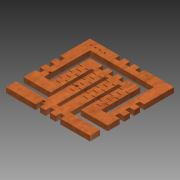
# Autodesk Inventor part: mech
Saved by Autodesk Inventor 2014 SP1 (Build 180222100, 222)
## iProperties
Created: 2015-02-17
Part Number: mech
Material: Wood (Cherry)
Document SubType Name: Modeling
Designer: Erin
Density: 0.63 g/cm^3
Appearance: Cherry - Natural Low Gloss
Author: Erin
Autodesk Inventor part; units mm, degrees
ref_plane "YZ Plane" through (0, 0, 0) normal (1, 0, 0) x (0, 1, 0)
ref_plane "XZ Plane" through (0, 0, 0) normal (0, 1, 0) x (-1, 0, 0)
ref_plane "XY Plane" through (0, 0, 0) normal (0, 0, 1) x (1, 0, 0)
sketch "slots" plane through (0, 0, 0) normal (0, 0, 1) x (1, 0, 0)
  line L0 (61.2067, 31.1821) -> (64.2567, 31.1821)
  line L1 (64.2567, 31.1821) -> (64.2567, 28.1071)
  line L2 (64.2567, 28.1071) -> (61.2067, 28.1071)
  line L3 (61.2067, 28.1071) -> (61.2067, 31.1821)
  line L4 (68.9317, 33.8834) -> (68.9317, 26.9198) construction
  line L5 (67.4067, 31.1821) -> (70.4567, 31.1821)
  line L6 (70.4567, 31.1821) -> (70.4567, 28.1071)
  line L7 (70.4567, 28.1071) -> (67.4067, 28.1071)
  line L8 (67.4067, 28.1071) -> (67.4067, 31.1821)
  line L9 (73.6067, 31.1821) -> (76.6567, 31.1821)
  line L10 (76.6567, 31.1821) -> (76.6567, 28.1071)
  line L11 (76.6567, 28.1071) -> (73.6067, 28.1071)
  line L12 (73.6067, 28.1071) -> (73.6067, 31.1821)
  line L13 (68.9317, 28.1071) -> (68.9317, 27.1937) construction
  point P0 (68.8645, 30.3856)
  dimension "d2" = 3.05
  dimension "d3" = 3.075
  dimension "d99" = 3.15
  dimension "d100" = 3.15
  measures "d2" distance of L1.end L2.end
  measures "d3" distance of L0.end L1.end
  measures "d99" distance between parallel lines of L8 L1
  measures "d100" distance between parallel lines of L12 L6
sketch "flexure" plane through (0, 0, 0) normal (0, 0, 1) x (1, 0, 0)
  line L0 (49.9032, 37.6477) -> (55.9032, 37.6477)
  line L1 (55.9032, 37.6477) -> (55.9032, 19.1477)
  line L2 (55.9032, 19.1477) -> (49.9032, 19.1477)
  line L3 (49.9032, 19.1477) -> (49.9032, 37.6477)
  line L4 (49.9032, 30.1477) -> (52.085, 30.1477)
  line L5 (52.085, 30.1477) -> (52.085, 29.6477)
  line L6 (52.085, 29.6477) -> (49.9032, 29.6477)
  line L7 (49.9032, 29.6477) -> (49.9032, 30.1477)
  line L8 (53.7214, 29.6477) -> (53.7214, 30.1477)
  line L9 (55.9032, 29.6477) -> (53.7214, 29.6477)
  line L10 (53.7214, 30.1477) -> (55.9032, 30.1477)
  line L11 (55.9032, 30.1477) -> (55.9032, 29.6477)
  line L12 (51.5395, 27.1477) -> (54.2668, 27.1477)
  line L13 (54.2668, 27.1477) -> (54.2668, 26.6477)
  line L14 (54.2668, 26.6477) -> (51.5395, 26.6477)
  line L15 (51.5395, 26.6477) -> (51.5395, 27.1477)
  line L16 (49.9032, 28.3977) -> (55.9032, 28.3977) construction
  line L17 (55.9032, 28.3977) -> (49.9032, 28.3977) construction
  line L18 (53.7214, 24.1477) -> (55.9032, 24.1477)
  line L19 (55.9032, 24.1477) -> (55.9032, 23.6477)
  line L20 (55.9032, 23.6477) -> (53.7214, 23.6477)
  line L21 (53.7214, 23.6477) -> (53.7214, 24.1477)
  line L22 (51.5395, 21.1477) -> (54.2668, 21.1477)
  line L23 (54.2668, 21.1477) -> (54.2668, 20.6477)
  line L24 (54.2668, 20.6477) -> (51.5395, 20.6477)
  line L25 (51.5395, 20.6477) -> (51.5395, 21.1477)
  line L26 (49.9032, 24.1477) -> (52.085, 24.1477)
  line L27 (52.085, 24.1477) -> (52.085, 23.6477)
  line L28 (52.085, 23.6477) -> (49.9032, 23.6477)
  line L29 (49.9032, 23.6477) -> (49.9032, 24.1477)
  line L30 (49.9032, 22.3977) -> (55.9032, 22.3977) construction
  line L31 (55.9032, 22.3977) -> (49.9032, 22.3977) construction
  line L32 (53.7214, 36.1477) -> (55.9032, 36.1477)
  line L33 (55.9032, 36.1477) -> (55.9032, 35.6477)
  line L34 (55.9032, 35.6477) -> (53.7214, 35.6477)
  line L35 (53.7214, 35.6477) -> (53.7214, 36.1477)
  line L36 (51.5395, 33.1477) -> (54.2668, 33.1477)
  line L37 (54.2668, 33.1477) -> (54.2668, 32.6477)
  line L38 (54.2668, 32.6477) -> (51.5395, 32.6477)
  line L39 (51.5395, 32.6477) -> (51.5395, 33.1477)
  line L40 (49.9032, 36.1477) -> (52.085, 36.1477)
  line L41 (52.085, 36.1477) -> (52.085, 35.6477)
  line L42 (52.085, 35.6477) -> (49.9032, 35.6477)
  line L43 (49.9032, 35.6477) -> (49.9032, 36.1477)
  line L44 (49.9032, 34.3977) -> (55.9032, 34.3977) construction
  line L45 (55.9032, 34.3977) -> (49.9032, 34.3977) construction
  line L46 (53.7214, 30.1477) -> (55.9032, 30.1477)
  line L47 (55.9032, 30.1477) -> (55.9032, 29.6477)
  line L48 (55.9032, 29.6477) -> (53.7214, 29.6477)
  line L49 (53.7214, 29.6477) -> (53.7214, 30.1477)
  line L50 (51.5395, 27.1477) -> (54.2668, 27.1477)
  line L51 (54.2668, 27.1477) -> (54.2668, 26.6477)
  line L52 (54.2668, 26.6477) -> (51.5395, 26.6477)
  line L53 (51.5395, 26.6477) -> (51.5395, 27.1477)
  line L54 (49.9032, 30.1477) -> (52.085, 30.1477)
  line L55 (52.085, 30.1477) -> (52.085, 29.6477)
  line L56 (52.085, 29.6477) -> (49.9032, 29.6477)
  line L57 (49.9032, 29.6477) -> (49.9032, 30.1477)
  line L58 (49.9032, 28.3977) -> (55.9032, 28.3977) construction
  line L59 (55.9032, 28.3977) -> (49.9032, 28.3977) construction
  line L60 (51.5395, 26.8977) -> (54.2668, 26.8977) construction
  point P0 (52.8239, 25.8216)
  dimension "d22" = 6
  dimension "d24" = 2.1818
  dimension "d27" = 3.8182
  dimension "d32" = 1.6364
  dimension "d33" = 2.7273
  dimension "d41" = 0.5
  dimension "d42" = 0.5
  dimension "d43" = 2.5
  dimension "d93" = 18.5
  dimension "d106" = 6
  dimension "d109" = 6
  dimension "d118" = 10.5
  measures "d22" distance of L1.end L2.end
  measures "d24" distance of L4.start L4.end
  measures "d27" distance of L6.end L9.end
  measures "d32" distance between parallel lines of L15 L3
  measures "d33" distance of L12.start L12.end
  measures "d41" distance of L4.end L5.end
  measures "d42" distance of L12.end L13.end
  measures "d43" distance between parallel lines of L12 L6
  measures "d93" distance of L0.end L1.end
  measures "d106" distance of L10.start L18.start
  measures "d109" distance of L10.start L32.start
  measures "d118" distance between parallel lines of L12 L0
sketch "Sketch1" plane through (0, 0, 0) normal (0, 0, 1) x (1, 0, 0)
  line L0 (-25, 25) -> (25, 25) construction
  line L1 (25, 25) -> (25, -25) construction
  line L2 (25, -25) -> (-25, -25) construction
  line L3 (-25, -25) -> (-25, 25) construction
  line L4 (-25, -25) -> (25, -25)
  line L5 (25, -25) -> (25, -19)
  line L6 (25, -19) -> (-25, -19)
  line L7 (-25, -19) -> (-25, -25)
  line L8 (0, 33.5916) -> (0, -39.9789) construction
  line L9 (-35.9054, 0) -> (42.6007, 0) construction
  line L10 (-25, 25) -> (25, 25)
  line L11 (25, 25) -> (25, 19)
  line L12 (25, 19) -> (-25, 19)
  line L13 (-25, 19) -> (-25, 25)
  line L14 (-25, 19) -> (-19, 19)
  line L15 (-19, 19) -> (-19, -14.5)
  line L16 (-19, -14.5) -> (-25, -14.5)
  line L17 (-25, -14.5) -> (-25, 19)
  line L18 (-19, -14.5) -> (-9, -14.5)
  line L19 (-9, -14.5) -> (-9, -8.5)
  line L20 (-9, -8.5) -> (-19, -8.5)
  line L21 (-19, -8.5) -> (-19, -14.5)
  line L22 (25, 19) -> (19, 19)
  line L23 (19, 19) -> (19, -14.5)
  line L24 (19, -14.5) -> (25, -14.5)
  line L25 (25, -14.5) -> (25, 19)
  line L26 (19, -14.5) -> (9, -14.5)
  line L27 (9, -14.5) -> (9, -8.5)
  line L28 (9, -8.5) -> (19, -8.5)
  line L29 (19, -8.5) -> (19, -14.5)
  line L30 (-15, 15) -> (15, 15)
  line L31 (15, 15) -> (15, 10)
  line L32 (15, 10) -> (-15, 10)
  line L33 (-15, 10) -> (-15, 15)
  line L34 (-7, -8.5) -> (-1, -8.5)
  line L35 (-1, -8.5) -> (-1, -19)
  line L36 (-1, -19) -> (-7, -19)
  line L37 (-7, -19) -> (-7, -8.5)
  line L38 (1, -8.5) -> (7, -8.5)
  line L39 (7, -8.5) -> (7, -19)
  line L40 (7, -19) -> (1, -19)
  line L41 (1, -19) -> (1, -8.5)
  line L42 (-68.1542, 16.5688) -> (-29.44, 16.5688) construction
  line L43 (-29.44, 16.5688) -> (-29.44, -5.0786) construction
  line L44 (-29.44, -5.0786) -> (-68.1542, -5.0786) construction
  line L45 (-68.1542, -5.0786) -> (-68.1542, 16.5688) construction
  circle A0 centre (-21.2866, 22) radius 0.5
  circle A1 centre (-18.6754, 22) radius 0.5
  circle A2 centre (-16, 22) radius 0.5
  circle A3 centre (-13.1389, 22) radius 0.5
  line L46 (-7.725, 25) -> (-4.675, 25)
  line L47 (-4.675, 25) -> (-4.675, 21.925)
  line L48 (-4.675, 21.925) -> (-7.725, 21.925)
  line L49 (-7.725, 21.925) -> (-7.725, 25)
  line L50 (0, 27.7013) -> (0, 20.7377) construction
  line L51 (-1.525, 25) -> (1.525, 25)
  line L52 (1.525, 25) -> (1.525, 21.925)
  line L53 (1.525, 21.925) -> (-1.525, 21.925)
  line L54 (-1.525, 21.925) -> (-1.525, 25)
  line L55 (4.675, 25) -> (7.725, 25)
  line L56 (7.725, 25) -> (7.725, 21.925)
  line L57 (7.725, 21.925) -> (4.675, 21.925)
  line L58 (4.675, 21.925) -> (4.675, 25)
  line L59 (0, 21.925) -> (0, 21.0116) construction
  line L60 (-7.725, -21.925) -> (-4.675, -21.925)
  line L61 (-4.675, -21.925) -> (-4.675, -25)
  line L62 (-4.675, -25) -> (-7.725, -25)
  line L63 (-7.725, -25) -> (-7.725, -21.925)
  line L64 (0, -19.2237) -> (0, -26.1873) construction
  line L65 (-1.525, -21.925) -> (1.525, -21.925)
  line L66 (1.525, -21.925) -> (1.525, -25)
  line L67 (1.525, -25) -> (-1.525, -25)
  line L68 (-1.525, -25) -> (-1.525, -21.925)
  line L69 (4.675, -21.925) -> (7.725, -21.925)
  line L70 (7.725, -21.925) -> (7.725, -25)
  line L71 (7.725, -25) -> (4.675, -25)
  line L72 (4.675, -25) -> (4.675, -21.925)
  line L73 (0, -25) -> (0, -25.9134) construction
  line L74 (-25, -7.725) -> (-25, -4.675)
  line L75 (-25, -4.675) -> (-21.925, -4.675)
  line L76 (-21.925, -4.675) -> (-21.925, -7.725)
  line L77 (-21.925, -7.725) -> (-25, -7.725)
  line L78 (-27.7013, 0) -> (-20.7377, 0) construction
  line L79 (-25, -1.525) -> (-25, 1.525)
  line L80 (-25, 1.525) -> (-21.925, 1.525)
  line L81 (-21.925, 1.525) -> (-21.925, -1.525)
  line L82 (-21.925, -1.525) -> (-25, -1.525)
  line L83 (-25, 4.675) -> (-25, 7.725)
  line L84 (-25, 7.725) -> (-21.925, 7.725)
  line L85 (-21.925, 7.725) -> (-21.925, 4.675)
  line L86 (-21.925, 4.675) -> (-25, 4.675)
  line L87 (-21.925, 0) -> (-21.0116, 0) construction
  line L88 (21.925, -7.725) -> (21.925, -4.675)
  line L89 (21.925, -4.675) -> (25, -4.675)
  line L90 (25, -4.675) -> (25, -7.725)
  line L91 (25, -7.725) -> (21.925, -7.725)
  line L92 (19.2237, 0) -> (26.1873, 0) construction
  line L93 (21.925, -1.525) -> (21.925, 1.525)
  line L94 (21.925, 1.525) -> (25, 1.525)
  line L95 (25, 1.525) -> (25, -1.525)
  line L96 (25, -1.525) -> (21.925, -1.525)
  line L97 (21.925, 4.675) -> (21.925, 7.725)
  line L98 (21.925, 7.725) -> (25, 7.725)
  line L99 (25, 7.725) -> (25, 4.675)
  line L100 (25, 4.675) -> (21.925, 4.675)
  line L101 (25, 0) -> (25.9134, 0) construction
  line L102 (-15, 10) -> (-9, 10)
  line L103 (-9, 10) -> (-9, -8.5)
  line L104 (-9, -8.5) -> (-15, -8.5)
  line L105 (-15, -8.5) -> (-15, 10)
  line L106 (-15, 2.5) -> (-12.8182, 2.5)
  line L107 (-12.8182, 2.5) -> (-12.8182, 2)
  line L108 (-12.8182, 2) -> (-15, 2)
  line L109 (-15, 2) -> (-15, 2.5)
  line L110 (-11.1818, 2) -> (-11.1818, 2.5)
  line L111 (-9, 2) -> (-11.1818, 2)
  line L112 (-11.1818, 2.5) -> (-9, 2.5)
  line L113 (-9, 2.5) -> (-9, 2)
  line L114 (-13.3636, -0.5) -> (-10.6364, -0.5)
  line L115 (-10.6364, -0.5) -> (-10.6364, -1)
  line L116 (-10.6364, -1) -> (-13.3636, -1)
  line L117 (-13.3636, -1) -> (-13.3636, -0.5)
  line L118 (-15, 0.75) -> (-9, 0.75) construction
  line L119 (-9, 0.75) -> (-15, 0.75) construction
  line L120 (-11.1818, -3.5) -> (-9, -3.5)
  line L121 (-9, -3.5) -> (-9, -4)
  line L122 (-9, -4) -> (-11.1818, -4)
  line L123 (-11.1818, -4) -> (-11.1818, -3.5)
  line L124 (-13.3636, -6.5) -> (-10.6364, -6.5)
  line L125 (-10.6364, -6.5) -> (-10.6364, -7)
  line L126 (-10.6364, -7) -> (-13.3636, -7)
  line L127 (-13.3636, -7) -> (-13.3636, -6.5)
  line L128 (-15, -3.5) -> (-12.8182, -3.5)
  line L129 (-12.8182, -3.5) -> (-12.8182, -4)
  line L130 (-12.8182, -4) -> (-15, -4)
  line L131 (-15, -4) -> (-15, -3.5)
  line L132 (-15, -5.25) -> (-9, -5.25) construction
  line L133 (-9, -5.25) -> (-15, -5.25) construction
  line L134 (-11.1818, 8.5) -> (-9, 8.5)
  line L135 (-9, 8.5) -> (-9, 8)
  line L136 (-9, 8) -> (-11.1818, 8)
  line L137 (-11.1818, 8) -> (-11.1818, 8.5)
  line L138 (-13.3636, 5.5) -> (-10.6364, 5.5)
  line L139 (-10.6364, 5.5) -> (-10.6364, 5)
  line L140 (-10.6364, 5) -> (-13.3636, 5)
  line L141 (-13.3636, 5) -> (-13.3636, 5.5)
  line L142 (-15, 8.5) -> (-12.8182, 8.5)
  line L143 (-12.8182, 8.5) -> (-12.8182, 8)
  line L144 (-12.8182, 8) -> (-15, 8)
  line L145 (-15, 8) -> (-15, 8.5)
  line L146 (-15, 6.75) -> (-9, 6.75) construction
  line L147 (-9, 6.75) -> (-15, 6.75) construction
  line L148 (-11.1818, 2.5) -> (-9, 2.5)
  line L149 (-9, 2.5) -> (-9, 2)
  line L150 (-9, 2) -> (-11.1818, 2)
  line L151 (-11.1818, 2) -> (-11.1818, 2.5)
  line L152 (-13.3636, -0.5) -> (-10.6364, -0.5)
  line L153 (-10.6364, -0.5) -> (-10.6364, -1)
  line L154 (-10.6364, -1) -> (-13.3636, -1)
  line L155 (-13.3636, -1) -> (-13.3636, -0.5)
  line L156 (-15, 2.5) -> (-12.8182, 2.5)
  line L157 (-12.8182, 2.5) -> (-12.8182, 2)
  line L158 (-12.8182, 2) -> (-15, 2)
  line L159 (-15, 2) -> (-15, 2.5)
  line L160 (-15, 0.75) -> (-9, 0.75) construction
  line L161 (-9, 0.75) -> (-15, 0.75) construction
  line L162 (-13.3636, -0.75) -> (-10.6364, -0.75) construction
  line L163 (9, 10) -> (15, 10)
  line L164 (15, 10) -> (15, -8.5)
  line L165 (15, -8.5) -> (9, -8.5)
  line L166 (9, -8.5) -> (9, 10)
  line L167 (9, 2.5) -> (11.1818, 2.5)
  line L168 (11.1818, 2.5) -> (11.1818, 2)
  line L169 (11.1818, 2) -> (9, 2)
  line L170 (9, 2) -> (9, 2.5)
  line L171 (12.8182, 2) -> (12.8182, 2.5)
  line L172 (15, 2) -> (12.8182, 2)
  line L173 (12.8182, 2.5) -> (15, 2.5)
  line L174 (15, 2.5) -> (15, 2)
  line L175 (10.6364, -0.5) -> (13.3636, -0.5)
  line L176 (13.3636, -0.5) -> (13.3636, -1)
  line L177 (13.3636, -1) -> (10.6364, -1)
  line L178 (10.6364, -1) -> (10.6364, -0.5)
  line L179 (9, 0.75) -> (15, 0.75) construction
  line L180 (15, 0.75) -> (9, 0.75) construction
  line L181 (12.8182, -3.5) -> (15, -3.5)
  line L182 (15, -3.5) -> (15, -4)
  line L183 (15, -4) -> (12.8182, -4)
  line L184 (12.8182, -4) -> (12.8182, -3.5)
  line L185 (10.6364, -6.5) -> (13.3636, -6.5)
  line L186 (13.3636, -6.5) -> (13.3636, -7)
  line L187 (13.3636, -7) -> (10.6364, -7)
  line L188 (10.6364, -7) -> (10.6364, -6.5)
  line L189 (9, -3.5) -> (11.1818, -3.5)
  line L190 (11.1818, -3.5) -> (11.1818, -4)
  line L191 (11.1818, -4) -> (9, -4)
  line L192 (9, -4) -> (9, -3.5)
  line L193 (9, -5.25) -> (15, -5.25) construction
  line L194 (15, -5.25) -> (9, -5.25) construction
  line L195 (12.8182, 8.5) -> (15, 8.5)
  line L196 (15, 8.5) -> (15, 8)
  line L197 (15, 8) -> (12.8182, 8)
  line L198 (12.8182, 8) -> (12.8182, 8.5)
  line L199 (10.6364, 5.5) -> (13.3636, 5.5)
  line L200 (13.3636, 5.5) -> (13.3636, 5)
  line L201 (13.3636, 5) -> (10.6364, 5)
  line L202 (10.6364, 5) -> (10.6364, 5.5)
  line L203 (9, 8.5) -> (11.1818, 8.5)
  line L204 (11.1818, 8.5) -> (11.1818, 8)
  line L205 (11.1818, 8) -> (9, 8)
  line L206 (9, 8) -> (9, 8.5)
  line L207 (9, 6.75) -> (15, 6.75) construction
  line L208 (15, 6.75) -> (9, 6.75) construction
  line L209 (12.8182, 2.5) -> (15, 2.5)
  line L210 (15, 2.5) -> (15, 2)
  line L211 (15, 2) -> (12.8182, 2)
  line L212 (12.8182, 2) -> (12.8182, 2.5)
  line L213 (10.6364, -0.5) -> (13.3636, -0.5)
  line L214 (13.3636, -0.5) -> (13.3636, -1)
  line L215 (13.3636, -1) -> (10.6364, -1)
  line L216 (10.6364, -1) -> (10.6364, -0.5)
  line L217 (9, 2.5) -> (11.1818, 2.5)
  line L218 (11.1818, 2.5) -> (11.1818, 2)
  line L219 (11.1818, 2) -> (9, 2)
  line L220 (9, 2) -> (9, 2.5)
  line L221 (9, 0.75) -> (15, 0.75) construction
  line L222 (15, 0.75) -> (9, 0.75) construction
  line L223 (10.6364, -0.75) -> (13.3636, -0.75) construction
  line L224 (1, 10) -> (7, 10)
  line L225 (7, 10) -> (7, -8.5)
  line L226 (7, -8.5) -> (1, -8.5)
  line L227 (1, -8.5) -> (1, 10)
  line L228 (1, 2.5) -> (3.1818, 2.5)
  line L229 (3.1818, 2.5) -> (3.1818, 2)
  line L230 (3.1818, 2) -> (1, 2)
  line L231 (1, 2) -> (1, 2.5)
  line L232 (4.8182, 2) -> (4.8182, 2.5)
  line L233 (7, 2) -> (4.8182, 2)
  line L234 (4.8182, 2.5) -> (7, 2.5)
  line L235 (7, 2.5) -> (7, 2)
  line L236 (2.6364, -0.5) -> (5.3636, -0.5)
  line L237 (5.3636, -0.5) -> (5.3636, -1)
  line L238 (5.3636, -1) -> (2.6364, -1)
  line L239 (2.6364, -1) -> (2.6364, -0.5)
  line L240 (1, 0.75) -> (7, 0.75) construction
  line L241 (7, 0.75) -> (1, 0.75) construction
  line L242 (4.8182, -3.5) -> (7, -3.5)
  line L243 (7, -3.5) -> (7, -4)
  line L244 (7, -4) -> (4.8182, -4)
  line L245 (4.8182, -4) -> (4.8182, -3.5)
  line L246 (2.6364, -6.5) -> (5.3636, -6.5)
  line L247 (5.3636, -6.5) -> (5.3636, -7)
  line L248 (5.3636, -7) -> (2.6364, -7)
  line L249 (2.6364, -7) -> (2.6364, -6.5)
  line L250 (1, -3.5) -> (3.1818, -3.5)
  line L251 (3.1818, -3.5) -> (3.1818, -4)
  line L252 (3.1818, -4) -> (1, -4)
  line L253 (1, -4) -> (1, -3.5)
  line L254 (1, -5.25) -> (7, -5.25) construction
  line L255 (7, -5.25) -> (1, -5.25) construction
  line L256 (4.8182, 8.5) -> (7, 8.5)
  line L257 (7, 8.5) -> (7, 8)
  line L258 (7, 8) -> (4.8182, 8)
  line L259 (4.8182, 8) -> (4.8182, 8.5)
  line L260 (2.6364, 5.5) -> (5.3636, 5.5)
  line L261 (5.3636, 5.5) -> (5.3636, 5)
  line L262 (5.3636, 5) -> (2.6364, 5)
  line L263 (2.6364, 5) -> (2.6364, 5.5)
  line L264 (1, 8.5) -> (3.1818, 8.5)
  line L265 (3.1818, 8.5) -> (3.1818, 8)
  line L266 (3.1818, 8) -> (1, 8)
  line L267 (1, 8) -> (1, 8.5)
  line L268 (1, 6.75) -> (7, 6.75) construction
  line L269 (7, 6.75) -> (1, 6.75) construction
  line L270 (4.8182, 2.5) -> (7, 2.5)
  line L271 (7, 2.5) -> (7, 2)
  line L272 (7, 2) -> (4.8182, 2)
  line L273 (4.8182, 2) -> (4.8182, 2.5)
  line L274 (2.6364, -0.5) -> (5.3636, -0.5)
  line L275 (5.3636, -0.5) -> (5.3636, -1)
  line L276 (5.3636, -1) -> (2.6364, -1)
  line L277 (2.6364, -1) -> (2.6364, -0.5)
  line L278 (1, 2.5) -> (3.1818, 2.5)
  line L279 (3.1818, 2.5) -> (3.1818, 2)
  line L280 (3.1818, 2) -> (1, 2)
  line L281 (1, 2) -> (1, 2.5)
  line L282 (1, 0.75) -> (7, 0.75) construction
  line L283 (7, 0.75) -> (1, 0.75) construction
  line L284 (2.6364, -0.75) -> (5.3636, -0.75) construction
  line L285 (-7, 10) -> (-1, 10)
  line L286 (-1, 10) -> (-1, -8.5)
  line L287 (-1, -8.5) -> (-7, -8.5)
  line L288 (-7, -8.5) -> (-7, 10)
  line L289 (-7, 2.5) -> (-4.8182, 2.5)
  line L290 (-4.8182, 2.5) -> (-4.8182, 2)
  line L291 (-4.8182, 2) -> (-7, 2)
  line L292 (-7, 2) -> (-7, 2.5)
  line L293 (-3.1818, 2) -> (-3.1818, 2.5)
  line L294 (-1, 2) -> (-3.1818, 2)
  line L295 (-3.1818, 2.5) -> (-1, 2.5)
  line L296 (-1, 2.5) -> (-1, 2)
  line L297 (-5.3636, -0.5) -> (-2.6364, -0.5)
  line L298 (-2.6364, -0.5) -> (-2.6364, -1)
  line L299 (-2.6364, -1) -> (-5.3636, -1)
  line L300 (-5.3636, -1) -> (-5.3636, -0.5)
  line L301 (-7, 0.75) -> (-1, 0.75) construction
  line L302 (-1, 0.75) -> (-7, 0.75) construction
  line L303 (-3.1818, -3.5) -> (-1, -3.5)
  line L304 (-1, -3.5) -> (-1, -4)
  line L305 (-1, -4) -> (-3.1818, -4)
  line L306 (-3.1818, -4) -> (-3.1818, -3.5)
  line L307 (-5.3636, -6.5) -> (-2.6364, -6.5)
  line L308 (-2.6364, -6.5) -> (-2.6364, -7)
  line L309 (-2.6364, -7) -> (-5.3636, -7)
  line L310 (-5.3636, -7) -> (-5.3636, -6.5)
  line L311 (-7, -3.5) -> (-4.8182, -3.5)
  line L312 (-4.8182, -3.5) -> (-4.8182, -4)
  line L313 (-4.8182, -4) -> (-7, -4)
  line L314 (-7, -4) -> (-7, -3.5)
  line L315 (-7, -5.25) -> (-1, -5.25) construction
  line L316 (-1, -5.25) -> (-7, -5.25) construction
  line L317 (-3.1818, 8.5) -> (-1, 8.5)
  line L318 (-1, 8.5) -> (-1, 8)
  line L319 (-1, 8) -> (-3.1818, 8)
  line L320 (-3.1818, 8) -> (-3.1818, 8.5)
  line L321 (-5.3636, 5.5) -> (-2.6364, 5.5)
  line L322 (-2.6364, 5.5) -> (-2.6364, 5)
  line L323 (-2.6364, 5) -> (-5.3636, 5)
  line L324 (-5.3636, 5) -> (-5.3636, 5.5)
  line L325 (-7, 8.5) -> (-4.8182, 8.5)
  line L326 (-4.8182, 8.5) -> (-4.8182, 8)
  line L327 (-4.8182, 8) -> (-7, 8)
  line L328 (-7, 8) -> (-7, 8.5)
  line L329 (-7, 6.75) -> (-1, 6.75) construction
  line L330 (-1, 6.75) -> (-7, 6.75) construction
  line L331 (-3.1818, 2.5) -> (-1, 2.5)
  line L332 (-1, 2.5) -> (-1, 2)
  line L333 (-1, 2) -> (-3.1818, 2)
  line L334 (-3.1818, 2) -> (-3.1818, 2.5)
  line L335 (-5.3636, -0.5) -> (-2.6364, -0.5)
  line L336 (-2.6364, -0.5) -> (-2.6364, -1)
  line L337 (-2.6364, -1) -> (-5.3636, -1)
  line L338 (-5.3636, -1) -> (-5.3636, -0.5)
  line L339 (-7, 2.5) -> (-4.8182, 2.5)
  line L340 (-4.8182, 2.5) -> (-4.8182, 2)
  line L341 (-4.8182, 2) -> (-7, 2)
  line L342 (-7, 2) -> (-7, 2.5)
  line L343 (-7, 0.75) -> (-1, 0.75) construction
  line L344 (-1, 0.75) -> (-7, 0.75) construction
  line L345 (-5.3636, -0.75) -> (-2.6364, -0.75) construction
  line L346 (-7.725, 15) -> (-4.675, 15)
  line L347 (-4.675, 15) -> (-4.675, 11.925)
  line L348 (-4.675, 11.925) -> (-7.725, 11.925)
  line L349 (-7.725, 11.925) -> (-7.725, 15)
  line L350 (0, 17.7013) -> (0, 10.7377) construction
  line L351 (-1.525, 15) -> (1.525, 15)
  line L352 (1.525, 15) -> (1.525, 11.925)
  line L353 (1.525, 11.925) -> (-1.525, 11.925)
  line L354 (-1.525, 11.925) -> (-1.525, 15)
  line L355 (4.675, 15) -> (7.725, 15)
  line L356 (7.725, 15) -> (7.725, 11.925)
  line L357 (7.725, 11.925) -> (4.675, 11.925)
  line L358 (4.675, 11.925) -> (4.675, 15)
  line L359 (0, 11.925) -> (0, 11.0116) construction
  point P0 (0, 0)
  point P1 (0, 25)
  point P2 (25, 0)
  point P3 (0, 15)
  point P4 (-4, -8.5)
  point P5 (-4, -8.5)
  point P6 (4, -8.5)
  point P7 (4, -8.5)
  dimension "d76" = 6
  dimension "d89" = 2
  dimension "d90" = 2
  dimension "d91" = 2
  dimension "d0" = 50
  dimension "d1" = 50
  dimension "d16" = 6
  dimension "d19" = 6
  dimension "d21" = 5
  dimension "d75" = 4
  dimension "d94" = 4
  dimension "d95" = 4.5
  dimension "d96" = 6
  dimension "d97" = 6
  dimension "d101" = 30
  dimension "d114" = 1
  dimension "d115" = 1
  dimension "d116" = 1
  dimension "d119" = 1
  constraints: 84 end point, 23 horizontal, 20 parallel, 11 perpendicular, 10 vertical, 5 equal length, 5 midpoint, 4 centre point, 3 collinear, 2 coincident, 2 point on line, 2 vertical alignment, 1 horizontal alignment, 4 other
  measures "d0" distance of L1.end L2.end
  measures "d1" distance of L0.end L1.end
  measures "d16" distance between parallel lines of L12 L10
  measures "d19" distance between parallel lines of L4 L6
  measures "d21" distance between parallel lines of L32 L30
  measures "d75" distance between parallel lines of L33 L15
  measures "d94" distance between parallel lines of L30 L12
  measures "d95" distance between parallel lines of L6 L16
  measures "d96" distance of L35.end L36.end
  measures "d97" distance of L39.end L40.end
  measures "d101" distance of L30.start L30.end
  measures "d114" diameter of A0
  measures "d115" diameter of A1
  measures "d116" diameter of A2
  measures "d119" diameter of A3
extrude "Extrusion3" add sketch "Sketch1" along normal blind 3.1 contours L7 L6 L5 L4 L70 L69 L72 L66 L65 L68 L61 L60 L63 | L37 L34 L35 L6 | L288 L313 L312 L311 L291 L290 L289 L327 L326 L325 L32 L286 L317 L320 L319 L295 L293 L294 L303 L306 L305 L34 | L41 L38 L39 L6 | L227 L252 L251 L250 L230 L229 L228 L266 L265 L264 L32 L225 L256 L259 L258 L234 L232 L233 L242 L245 L244 L38 | L32 L33 L30 L349 L348 L347 L354 L353 L352 L358 L357 L356 L31 | L103 L134 L137 L136 L112 L110 L111 L120 L123 L122 L20 L105 L130 L129 L128 L108 L107 L106 L144 L143 L142 L32 | L32 L164 L195 L198 L197 L173 L171 L172 L181 L184 L183 L28 L166 L191 L190 L189 L169 L168 L167 L205 L204 L203 | L19 L18 L15 L20 | L15 L16 L17 L77 L76 L75 L82 L81 L80 L86 L85 L84 L12 | L28 L23 L26 L27 | L12 L13 L10 L49 L48 L47 L54 L53 L52 L58 L57 L56 L11 | L12 L25 L98 L97 L100 L94 L93 L96 L89 L88 L91 L24 L23
equation "\"d2\" = mat - kerf"
equation "\"d3\" = mat - 0.5 * kerf"
equation "\"d22\" = flex_w"
equation "\"d24\" = 0.363636 * flex_w"
equation "\"d27\" = 0.636364 * flex_w"
equation "\"d32\" = 0.272727 * flex_w"
equation "\"d33\" = 0.454545 * flex_w"
equation "\"d41\" = line_w"
equation "\"d42\" = line_w"
equation "\"d43\" = line_sp"
equation "\"d93\" = flex_h"
equation "\"d89\" = flex_sp"
equation "\"d90\" = flex_sp"
equation "\"d16\" = structure_w"
equation "\"d19\" = structure_w"
equation "\"structure_w\" = 6"
equation "\"structure_sp\" = 8"
equation "\"flex_w\" = 6"
equation "\"flex_h\" = 18.5"
equation "\"line_w\" = 0.5"
equation "\"line_sp\" = 2.5"
equation "\"flex_sp\" = 2"
equation "\"mat\" = 3.1"
equation "\"kerf\" = 0.05"
body "Solid3"
